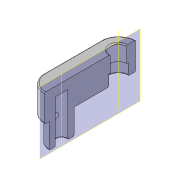
# Autodesk Inventor part: replacementHandleStuipt
Saved by Autodesk Inventor 2021 (Build 250183000, 183)
## iProperties
Created: 2020-07-30
Part Number: replacementHandleStuipt
Material: Generic
Document SubType Name: Modeling
Designer: Stu
Density: 1 g/cm^3
Appearance: Default
Author: Stu
Autodesk Inventor part; units mm, degrees
ref_plane "YZ Plane" through (0, 0, 0) normal (1, 0, 0) x (0, 1, 0)
ref_plane "XZ Plane" through (0, 0, 0) normal (0, 1, 0) x (-1, 0, 0)
ref_plane "XY Plane" through (0, 0, 0) normal (0, 0, 1) x (1, 0, 0)
sketch "Sketch1" plane through (0, 0, 0) normal (0, 1, 0) x (-1, 0, 0)
  line L0 (0, 0) -> (58.9699, 0) construction
  line L1 (0, 0) -> (-34.9844, 0) construction
  line L2 (54.4643, -50) -> (-40.1402, -50) construction
  line L3 (0, 6.721) -> (0, -67.757)
  arc A0 (15, 0) -> (-15, 0) centre (0, 0) ccw
  arc A1 (-15, -50) -> (15, -50) centre (0, -50) ccw
  line L4 (-15, -50) -> (-15, 0)
  line L5 (15, -50) -> (15, 0)
  dimension "d7" = 50
  dimension "d8" = 15
  dimension "d9" = 15
  constraints: 12 end point, 7 point on line, 5 point on circle, 2 centre point, 2 horizontal, 1 coincident, 1 parallel, 1 vertical
  measures "d7" distance between parallel lines of L2 L0
  measures "d8" radius of A0
  measures "d9" radius of A1
extrude "Extrusion1" add sketch "Sketch1" along normal blind 24
sketch "Sketch2" plane through (0, 0, 0) normal (0, -1, 0) x (1, 0, 0)
  circle A0 centre (0, 0) radius 11
  dimension "d12" = 22
  constraints: 1 centre point, 1 coincident
  measures "d12" diameter of A0
extrude "Extrusion2" add sketch "Sketch2" along normal blind 22
sketch "Sketch8" plane through (0, -22, 0) normal (0, -1, 0) x (1, 0, 0)
  circle A0 centre (0, 0) radius 5.5
  dimension "d26" = 11
  constraints: 1 centre point, 1 coincident
  measures "d26" diameter of A0
extrude "Extrusion6" cut sketch "Sketch8" against normal blind 38.1
sketch "Sketch10" plane through (0, 24, 0) normal (0, 1, 0) x (1, 0, 0)
  line L0 (0, 0) -> (0, 50) construction
  circle A0 centre (0, 50) radius 8.5
  dimension "d38" = 50
  dimension "d39" = 17
  constraints: 2 end point, 1 centre point, 1 coincident, 1 vertical
  measures "d38" distance of L0.start L0.end
  measures "d39" diameter of A0
extrude "Extrusion8" cut sketch "Sketch10" against normal through all
sketch "Sketch11" plane through (0, 24, 0) normal (0, 1, 0) x (1, 0, 0)
  circle A0 centre (0, 50) radius 8.5 projected
  circle A1 centre (0, 50) radius 8.5
  circle A2 centre (0, 50) radius 7.25
  point P0 (0, 0)
  dimension "d42" = 14.5
  constraints: 2 centre point, 2 coincident, 1 concentric
  measures "d42" diameter of A2
extrude "Extrusion9" add sketch "Sketch11" against normal blind 14
ref_plane "Work Plane1" through (0, -22, 0) normal (-1, 0, 0) x (0, 1, 0)
sketch "Sketch9" plane through (0, -22, 0) normal (-1, 0, 0) x (0, 1, 0)
  line L0 (0, 11) -> (0, -11) construction
  line L1 (0, -11) -> (24, -11) construction
  line L2 (24, -11) -> (24, 11) construction
  line L3 (24, 11) -> (0, 11) construction
  line L4 (0, 11) -> (0, -11) construction
  line L5 (0, -5.5) -> (0, 5.5) construction
  line L6 (0, 0) -> (18, 0) construction
  circle A0 centre (18, 0) radius 2.5
  point P0 (22, 0)
  dimension "d33" = 18
  dimension "d34" = 5
  constraints: 10 end point, 2 horizontal, 2 parallel, 1 centre point, 1 coincident, 1 midpoint, 1 perpendicular
  measures "d33" distance of L6.start L6.end
  measures "d34" diameter of A0
extrude "Extrusion7" cut sketch "Sketch9" along normal through all both and the other way through all
fillet "Fillet1" radius 1 14 edges at (15, 24, -25) (-15, 24, -25) (0, 24, 15) (-5.5, -22, 0) (0, 0, 15) (15, 0, -25) (0, 0, -65) (-15, 0, -25) (10.7121, -3.9998, -2.5) (10.7121, -4.0003, 2.5) (-11, -6.5, 0.0006) (-11, -22, 0) (-7.25, 24, -50) (-8.5, 0, -50)
sketch "Sketch12" plane through (0, -22, 0) normal (-1, 0, 0) x (0, 1, 0)
  line L0 (50.4549, -17.897) -> (-1.3047, -17.897)
  line L1 (-1.3047, -17.897) -> (-1.3047, 67.7253)
  line L2 (-1.3047, 67.7253) -> (50.4549, 67.7253)
  line L3 (50.4549, 67.7253) -> (50.4549, -17.897)
  point P0 (22, 0)
  constraints: 8 end point, 2 parallel, 1 horizontal, 1 perpendicular
extrude "Extrusion10" [suppressed]
body "Solid1"
